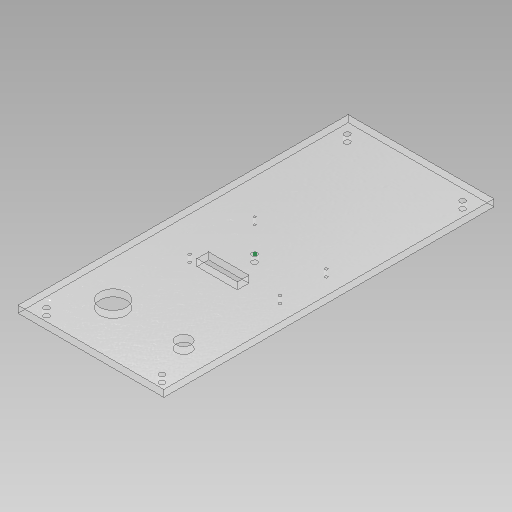
# Autodesk Inventor part: platform_plate
Saved by Autodesk Inventor 2020 (Build 240168000, 168)
## iProperties
Created: 2022-08-12
Part Number: platform_plate
Material: Acrylic
Document SubType Name: Modeling
Designer: Umair
Density: 1.188 g/cm^3
Appearance: Transparent - Clear
Author: Umair
Autodesk Inventor part; units mm, degrees
ref_plane "YZ Plane" through (0, 0, 0) normal (1, 0, 0) x (0, 1, 0)
ref_plane "XZ Plane" through (0, 0, 0) normal (0, 1, 0) x (-1, 0, 0)
ref_plane "XY Plane" through (0, 0, 0) normal (0, 0, 1) x (1, 0, 0)
sketch "Sketch1" plane through (0, 0, 0) normal (0, 1, 0) x (-1, 0, 0)
  line L0 (50, 130) -> (-50, 130)
  line L1 (-50, 130) -> (-50, -130)
  line L2 (-50, -130) -> (50, -130)
  line L3 (50, -130) -> (50, 130)
  line L4 (50, 130) -> (-50, -130) construction
  line L5 (-50, 130) -> (50, -130) construction
  line L6 (57.5, 137.5) -> (-57.5, 137.5)
  line L7 (-57.5, 137.5) -> (-57.5, -137.5)
  line L8 (-57.5, -137.5) -> (57.5, -137.5)
  line L9 (57.5, -137.5) -> (57.5, 137.5)
  line L10 (57.5, 137.5) -> (-57.5, -137.5) construction
  line L11 (-57.5, 137.5) -> (57.5, -137.5) construction
  circle A0 centre (50, 130) radius 2.5
  circle A1 centre (-50, 130) radius 2.5
  circle A2 centre (-50, -130) radius 2.5
  circle A3 centre (50, -130) radius 2.5
  point P0 (0, 0)
  dimension "d0" = 100
  dimension "d1" = 260
  dimension "d2" = 115
  dimension "d3" = 275
  dimension "d4" = 5
  dimension "d5" = 5
  dimension "d6" = 5
  dimension "d7" = 5
  constraints: 24 end point, 4 centre point, 4 coincident, 4 midpoint, 4 parallel, 2 horizontal, 2 perpendicular
  measures "d0" distance of L2.end L1.end
  measures "d1" distance of L1.end L0.end
  measures "d2" distance of L8.end L7.end
  measures "d3" distance of L7.end L6.end
  measures "d4" diameter of A0
  measures "d5" diameter of A1
  measures "d6" diameter of A2
  measures "d7" diameter of A3
extrude "Extrusion1" add sketch "Sketch1" along normal blind 6 contours L0 A0 L3 A3 L2 A2 L1 A1 | L9 L8 L7 L6
sketch "Sketch2" plane through (0, 6, 0) normal (0, 1, 0) x (1, 0, 0)
  circle A0 centre (0, 0) radius 2.5
  line L0 (0, 0) -> (42, 0)
  line L1 (42, 0) -> (0, 0)
  line L2 (0, 0) -> (-28, 0)
  line L3 (-28, 0) -> (-28, 28)
  line L4 (-28, 28) -> (-28, -28)
  line L5 (42, 0) -> (42, 20)
  line L6 (42, 20) -> (42, -20)
  circle A1 centre (-28, -28) radius 1.25
  circle A2 centre (-28, 28) radius 1
  circle A3 centre (42, 20) radius 1.25
  circle A4 centre (42, -20) radius 1.25
  line L7 (-21.6952, -23.1643) -> (-21.6952, -28.1643)
  line L8 (-21.6952, -28.1643) -> (-21.6952, -23.1643)
  line L9 (-21.6952, -23.1643) -> (-21.6952, -18.1643)
  line L10 (-21.6952, -18.1643) -> (13.3048, -18.1643)
  line L11 (13.3048, -18.1643) -> (13.3048, -28.1643)
  line L12 (13.3048, -28.1643) -> (-21.6952, -28.1643)
  dimension "d10" = 5
  dimension "d11" = 42
  dimension "d12" = 42
  dimension "d13" = 28
  dimension "d14" = 28
  dimension "d15" = 56
  dimension "d16" = 20
  dimension "d17" = 40
  dimension "d18" = 2.5
  dimension "d19" = 2
  dimension "d20" = 2.5
  dimension "d21" = 2.5
  dimension "d22" = 5
  dimension "d23" = 5
  dimension "d24" = 5
  dimension "d25" = 35
  constraints: 26 end point, 5 centre point, 5 coincident, 4 perpendicular, 4 point on line, 2 collinear, 1 horizontal, 1 vertical
  measures "d10" diameter of A0
  measures "d11" distance of L0.start L0.end
  measures "d12" distance of L0.end L0.start
  measures "d13" distance of L0.start L2.end
  measures "d14" distance of L2.end L3.end
  measures "d15" distance of L3.end L4.end
  measures "d16" distance of L0.end L5.end
  measures "d17" distance of L5.end L6.end
  measures "d18" diameter of A1
  measures "d19" diameter of A2
  measures "d20" diameter of A3
  measures "d21" diameter of A4
  measures "d22" distance of L7.start L7.end
  measures "d23" distance of L7.end L7.start
  measures "d24" distance of L7.start L9.end
  measures "d25" distance of L9.end L10.end
extrude "Extrusion2" cut sketch "Sketch2" against normal blind 6
sketch "Sketch3" plane through (0, 6, 0) normal (0, 1, 0) x (1, 0, 0)
  point P0 (0, 0)
sketch "Sketch4" plane through (0, 6, 0) normal (0, 1, 0) x (1, 0, 0)
  line L0 (-57.5, 137.5) -> (-57.5, -137.5) projected
  line L1 (-57.5, -137.5) -> (-57.5, 0)
  line L2 (-21.6952, -18.1643) -> (-21.6952, -28.1643) projected
  line L3 (-21.6952, -28.1643) -> (-75.3295, -28.1643)
  line L4 (-75.3295, -28.1643) -> (-57.5, -28.1643)
  line L5 (-57.5, -137.5) -> (-57.5, -28.1643)
  line L6 (-57.5, -28.1643) -> (-57.5, -82.8322)
  line L7 (-57.5, -82.8322) -> (-27.1083, -82.8322)
  line L8 (-27.1083, -82.8322) -> (0, -82.8322)
  line L9 (0, -82.8322) -> (72.7953, -82.8322)
  line L10 (72.7953, -82.8322) -> (0, -82.8322)
  line L11 (0, -95.2871) -> (0, -82.8322)
  line L12 (0, -95.2871) -> (-27.1083, -95.2871)
  line L13 (-27.1083, -95.2871) -> (0, -95.2871)
  line L14 (33.9195, -95.2871) -> (0, -95.2871)
  circle A0 centre (-27.1083, -95.2871) radius 11.5
  circle A1 centre (33.9195, -95.2871) radius 6.5
  point P0 (0, 0)
  dimension "d28" = 23
  dimension "d29" = 13
  constraints: 26 end point, 5 point on line, 3 collinear, 3 horizontal, 2 centre point, 2 coincident, 2 midpoint, 2 perpendicular
  measures "d28" diameter of A0
  measures "d29" diameter of A1
extrude "Extrusion3" cut sketch "Sketch4" against normal blind 10
sketch "Sketch5" plane through (0, 6, 0) normal (0, 1, 0) x (1, 0, 0)
  line L0 (-57.5, -137.5) -> (57.5, -137.5) projected
  line L1 (-57.5, -137.5) -> (-64.1, -137.5)
  line L2 (57.5, 137.5) -> (-57.5, 137.5) projected
  line L3 (-57.5, 137.5) -> (-64.1, 137.5)
  line L4 (-64.1, 137.5) -> (-64.1, -137.5)
  line L5 (-64.1, 137.5) -> (-64.1, 145)
  line L6 (-64.1, 145) -> (57.5, 145)
  line L7 (57.5, 145) -> (57.5, 137.5)
  line L8 (57.5, 145) -> (62, 145)
  line L9 (62, 145) -> (62, -137.5)
  line L10 (57.5, -137.5) -> (57.5, 137.5) projected
  line L11 (62, -137.5) -> (57.5, -137.5)
  line L12 (-64.1, -137.5) -> (-64.1, -140.5)
  line L13 (-64.1, -140.5) -> (62, -140.5)
  line L14 (62, -140.5) -> (62, -137.5)
  line L15 (-57.5, -137.5) -> (-57.5, 137.5)
  line L16 (57.5, 137.5) -> (57.5, -137.5)
  point P0 (0, 0)
  dimension "d32" = 6.6
  dimension "d33" = 6.6
  dimension "d34" = 7.5
  dimension "d35" = 4.5
  dimension "d36" = 3
  constraints: 28 end point, 5 perpendicular, 3 horizontal, 2 vertical, 1 collinear, 1 parallel, 1 point on line
  measures "d32" distance of L0.start L1.end
  measures "d33" distance of L2.end L3.end
  measures "d34" distance of L3.end L5.end
  measures "d35" distance of L6.end L8.end
  measures "d36" distance of L1.end L12.end
extrude "Extrusion4" add sketch "Sketch5" against normal blind 6 contours L0 L11 L14 L13 L12 L1 | L1 L4 L3 L15 | L10 L7 L8 L9 L11 | L3 L5 L6 L7 L2
body "Solid1"
